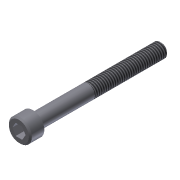
# Autodesk Inventor part: 10-32 x1000
Saved by Autodesk Inventor 2011 SP1 (Build 150282100, 282)
## iProperties
Created: 2011-07-11
Part Number: 10-32 x1000
Document SubType Name: Modeling
Designer: Dan Niemitalo
Density: 7.85 g/cm^3
Material: Steel
Mass: 7.87296 g
Surface Area: 9.2378 cm^2
Volume: 1.00292 cm^3
Author: Dan Niemitalo
Autodesk Inventor part; units mm, degrees
ref_plane "YZ Plane" through (0, 0, 0) normal (1, 0, 0) x (0, 1, 0)
ref_plane "XZ Plane" through (0, 0, 0) normal (0, 1, 0) x (-1, 0, 0)
ref_plane "XY Plane" through (0, 0, 0) normal (0, 0, 1) x (1, 0, 0)
sketch "Sketch1" plane through (0, 0, 0) normal (0, 0, 1) x (1, 0, 0)
  circle A0 centre (0, 0) radius 3.9624
  dimension "d0" = 7.9248
  constraints: 1 centre point, 1 coincident
  measures "d0" diameter of A0
extrude "Extrusion1" add sketch "Sketch1" along normal blind 4.826
sketch "Sketch2" plane through (0, 0, 0) normal (0, 0, -1) x (-1, 0, 0)
  circle A0 centre (0, 0) radius 3.9624 projected
  circle A1 centre (0, 0) radius 2.413
  dimension "d3" = 4.826
  constraints: 1 centre point, 1 coincident
  measures "d3" diameter of A1
extrude "Extrusion2" add sketch "Sketch2" along normal blind 44.45 contours A1
sketch "Sketch3" plane through (0, 0, 4.826) normal (0, 0, 1) x (1, 0, 0)
  circle A0 centre (0, 0) radius 3.9624 projected
  line L0 (-1.1457, 1.9844) -> (1.1457, 1.9844)
  line L1 (1.1457, 1.9844) -> (2.2914, 0)
  line L2 (2.2914, 0) -> (1.1457, -1.9844)
  line L3 (1.1457, -1.9844) -> (-1.1457, -1.9844)
  line L4 (-1.1457, -1.9844) -> (-2.2914, 0)
  line L5 (-2.2914, 0) -> (-1.1457, 1.9844)
  dimension "d6" = 3.9688
  constraints: 12 end point, 1 coincident, 1 horizontal, 13 other
  measures "d6" distance between parallel lines of L3 L0
extrude "Extrusion3" cut sketch "Sketch3" against normal blind 3.175 contours L0 L1 L2 L3 L4 L5
thread "Thread1" size "10-32 UNF" class "2A" standard "ANSI Unified Screw Threads" length 25.4
chamfer "Chamfer1" distance 0.508 angle 45 1 edges at (2.413, 0, -44.45)
chamfer "Chamfer2" distance 0.508 angle 45 1 edges at (-3.9624, 0, 4.826)
body "Solid1"
